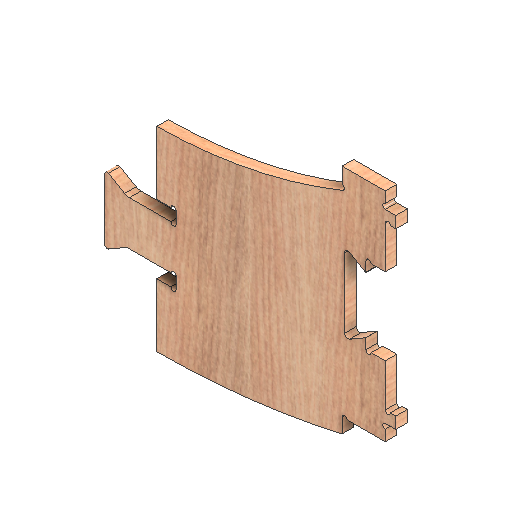
# Autodesk Inventor part: Support C
Saved by Autodesk Inventor 2021 (Build 250183000, 183)
## iProperties
Created: 2020-05-09
Part Number: Support C
Material: Wood (Birch)
Document SubType Name: Modeling
Designer: Dan Wikman
Density: 0.55 g/cm^3
Appearance: Birch - Natural Polished
Mass: 1099.51 g
Surface Area: 2585.2 cm^2
Volume: 1999.1 cm^3
Autodesk Inventor part; units mm, degrees
ref_plane "YZ Plane" through (0, 0, 0) normal (1, 0, 0) x (0, 1, 0)
ref_plane "XZ Plane" through (0, 0, 0) normal (0, 1, 0) x (-1, 0, 0)
ref_plane "XY Plane" through (0, 0, 0) normal (0, 0, 1) x (1, 0, 0)
sketch "CONTOURS" plane through (0, 0, 0) normal (0, 0, 1) x (1, 0, 0)
  arc A0 (167.5054, 852.7989) -> (159.5054, 852.7989) centre (163.5054, 852.7989) ccw
  line L0 (159.5054, 852.7989) -> (95.0246, 852.7989)
  arc A1 (95.0246, 852.7989) -> (87.5246, 850.7893) centre (95.0246, 837.7989) ccw
  line L1 (87.5246, 850.7893) -> (62.3643, 836.263)
  arc A2 (56.3643, 839.7271) -> (62.3643, 836.263) centre (60.3643, 839.7271) ccw
  line L2 (56.3643, 839.7271) -> (56.3643, 934.8707)
  arc A3 (62.3643, 938.3348) -> (56.3643, 934.8707) centre (60.3643, 934.8707) ccw
  line L3 (62.3643, 938.3348) -> (87.5246, 923.8085)
  arc A4 (87.5246, 923.8085) -> (95.0246, 921.7989) centre (95.0246, 936.7989) ccw
  line L4 (95.0246, 921.7989) -> (136.0054, 921.7989)
  line L5 (136.0054, 921.7989) -> (159.5054, 921.7989)
  arc A5 (159.5054, 921.7989) -> (167.5054, 921.7989) centre (163.5054, 921.7989) ccw
  line L6 (167.5054, 921.7989) -> (167.5054, 940.7989)
  arc A6 (167.5054, 940.7989) -> (159.5054, 940.7989) centre (163.5054, 940.7989) ccw
  line L7 (159.5054, 940.7989) -> (137.5054, 940.7989)
  line L8 (137.5054, 940.7989) -> (137.5054, 1039.1352)
  arc A7 (137.5054, 1039.1352) -> (426.0054, 1097.3015) centre (128.2106, 1829.7885) ccw
  arc A8 (426.0054, 1097.3015) -> (426.0054, 1105.3015) centre (426.0054, 1101.3015) ccw
  line L9 (426.0054, 1105.3015) -> (426.0054, 1129.8557)
  line L10 (426.0054, 1129.8557) -> (493.1464, 1129.8556)
  line L11 (493.1464, 1129.8556) -> (493.1464, 1113.0556)
  arc A9 (493.1464, 1113.0556) -> (493.1464, 1105.0556) centre (493.1464, 1109.0556) ccw
  line L12 (493.1464, 1105.0556) -> (509.6464, 1105.0556)
  line L13 (509.6464, 1105.0556) -> (509.6464, 1087.0556)
  line L14 (509.6464, 1087.0556) -> (501.1464, 1087.0556)
  arc A10 (501.1464, 1087.0556) -> (493.1464, 1087.0556) centre (497.1464, 1087.0556) ccw
  line L15 (493.1464, 1087.0556) -> (493.1464, 1020.8556)
  line L16 (493.1464, 1020.8556) -> (471.1464, 1020.8556)
  arc A11 (471.1464, 1020.8556) -> (463.1464, 1020.8556) centre (467.1464, 1020.8556) ccw
  line L17 (463.1464, 1020.8556) -> (463.1464, 1004.6734)
  line L18 (463.1464, 1004.6734) -> (462.9047, 1004.8036)
  line L19 (462.9047, 1004.8036) -> (462.6656, 1004.9385)
  line L20 (462.6656, 1004.9385) -> (437.5054, 1019.4648)
  arc A12 (437.5054, 1019.4648) -> (430.0054, 1015.1347) centre (435.0054, 1015.1347) ccw
  line L21 (430.0054, 1015.1347) -> (430.0054, 906.5765)
  arc A13 (430.0054, 906.5765) -> (437.5054, 902.2464) centre (435.0054, 906.5765) ccw
  line L22 (437.5054, 902.2464) -> (462.6656, 916.7727)
  line L23 (462.6656, 916.7727) -> (462.9047, 916.9076)
  line L24 (462.9047, 916.9076) -> (463.1464, 917.0378)
  line L25 (463.1464, 917.0378) -> (463.1464, 900.8556)
  arc A14 (463.1464, 900.8556) -> (471.1464, 900.8556) centre (467.1464, 900.8556) ccw
  line L26 (471.1464, 900.8556) -> (493.1464, 900.8556)
  line L27 (493.1464, 900.8556) -> (493.1464, 834.6556)
  arc A15 (493.1464, 834.6556) -> (501.1464, 834.6556) centre (497.1464, 834.6556) ccw
  line L28 (501.1464, 834.6556) -> (509.6464, 834.6556)
  line L29 (509.6464, 834.6556) -> (509.6464, 816.6556)
  line L30 (509.6464, 816.6556) -> (493.1464, 816.6556)
  arc A16 (493.1464, 816.6556) -> (493.1464, 808.6556) centre (493.1464, 812.6556) ccw
  line L31 (493.1464, 808.6556) -> (493.1464, 791.8557)
  line L32 (493.1464, 791.8557) -> (434.0054, 791.8557)
  arc A17 (434.0054, 791.8557) -> (426.0054, 791.8557) centre (430.0054, 791.8557) ccw
  line L33 (426.0054, 791.8557) -> (426.0054, 768.8809)
  arc A18 (137.5054, 735.4635) -> (426.0054, 768.8809) centre (133.6317, 2030.9546) ccw
  line L34 (137.5054, 735.4635) -> (137.5054, 833.7989)
  line L35 (137.5054, 833.7989) -> (159.5054, 833.7989)
  arc A19 (159.5054, 833.7989) -> (167.5054, 833.7989) centre (163.5054, 833.7989) ccw
  line L36 (167.5054, 833.7989) -> (167.5054, 852.7989)
  constraints: 74 end point, 40 point on circle, 20 centre point
sketch "LETTERS" plane through (0, 0, 0) normal (0, 0, 1) x (1, 0, 0)
  line L0 (285.7416, 916.5238) -> (285.9594, 916.4912)
  line L1 (285.9594, 916.4912) -> (286.1742, 916.4519)
  line L2 (286.1742, 916.4519) -> (286.386, 916.4061)
  line L3 (286.386, 916.4061) -> (286.5947, 916.3537)
  line L4 (286.5947, 916.3537) -> (286.8003, 916.2951)
  line L5 (286.8003, 916.2951) -> (287.0028, 916.2304)
  line L6 (287.0028, 916.2304) -> (287.2021, 916.1595)
  line L7 (287.2021, 916.1595) -> (287.3982, 916.0828)
  line L8 (287.3982, 916.0828) -> (287.5911, 916.0003)
  line L9 (287.5911, 916.0003) -> (287.7807, 915.9122)
  line L10 (287.7807, 915.9122) -> (287.967, 915.8185)
  line L11 (287.967, 915.8185) -> (288.1499, 915.7195)
  line L12 (288.1499, 915.7195) -> (288.3295, 915.6152)
  line L13 (288.3295, 915.6152) -> (288.5057, 915.5058)
  line L14 (288.5057, 915.5058) -> (288.6784, 915.3914)
  line L15 (288.6784, 915.3914) -> (288.8477, 915.2722)
  line L16 (288.8477, 915.2722) -> (289.0135, 915.1482)
  line L17 (289.0135, 915.1482) -> (289.1757, 915.0197)
  line L18 (289.1757, 915.0197) -> (289.3343, 914.8867)
  line L19 (289.3343, 914.8867) -> (289.4894, 914.7494)
  line L20 (289.4894, 914.7494) -> (289.6408, 914.6079)
  line L21 (289.6408, 914.6079) -> (289.7885, 914.4624)
  line L22 (289.7885, 914.4624) -> (289.9325, 914.3129)
  line L23 (289.9325, 914.3129) -> (290.0728, 914.1596)
  line L24 (290.0728, 914.1596) -> (290.2093, 914.0027)
  line L25 (290.2093, 914.0027) -> (290.3419, 913.8423)
  line L26 (290.3419, 913.8423) -> (290.4708, 913.6784)
  line L27 (290.4708, 913.6784) -> (290.5957, 913.5113)
  line L28 (290.5957, 913.5113) -> (290.7168, 913.3411)
  line L29 (290.7168, 913.3411) -> (290.8339, 913.1679)
  line L30 (290.8339, 913.1679) -> (290.947, 912.9918)
  line L31 (290.947, 912.9918) -> (291.0561, 912.813)
  line L32 (291.0561, 912.813) -> (291.1611, 912.6315)
  line L33 (291.1611, 912.6315) -> (291.2621, 912.4476)
  line L34 (291.2621, 912.4476) -> (291.359, 912.2614)
  line L35 (291.359, 912.2614) -> (291.4517, 912.073)
  line L36 (291.4517, 912.073) -> (291.5402, 911.8825)
  line L37 (291.5402, 911.8825) -> (291.6245, 911.69)
  line L38 (291.6245, 911.69) -> (291.7046, 911.4958)
  line L39 (291.7046, 911.4958) -> (291.7803, 911.2999)
  line L40 (291.7803, 911.2999) -> (291.8518, 911.1024)
  line L41 (291.8518, 911.1024) -> (291.9189, 910.9035)
  line L42 (291.9189, 910.9035) -> (291.9816, 910.7034)
  line L43 (291.9816, 910.7034) -> (292.0399, 910.5021)
  line L44 (292.0399, 910.5021) -> (292.0938, 910.2998)
  line L45 (292.0938, 910.2998) -> (292.1431, 910.0966)
  line L46 (292.1431, 910.0966) -> (292.1879, 909.8927)
  line L47 (292.1879, 909.8927) -> (292.2282, 909.6881)
  line L48 (292.2282, 909.6881) -> (292.2639, 909.4831)
  line L49 (292.2639, 909.4831) -> (292.295, 909.2777)
  line L50 (292.295, 909.2777) -> (292.3214, 909.0721)
  line L51 (292.3214, 909.0721) -> (292.3431, 908.8665)
  line L52 (292.3431, 908.8665) -> (292.3601, 908.6608)
  line L53 (292.3601, 908.6608) -> (292.3724, 908.4554)
  line L54 (292.3724, 908.4554) -> (292.3798, 908.2502)
  line L55 (292.3798, 908.2502) -> (292.3825, 908.0455)
  line L56 (292.3825, 908.0455) -> (292.3802, 907.8414)
  line L57 (292.3802, 907.8414) -> (292.3731, 907.638)
  line L58 (292.3731, 907.638) -> (292.3611, 907.4354)
  line L59 (292.3611, 907.4354) -> (292.3441, 907.2338)
  line L60 (292.3441, 907.2338) -> (292.3221, 907.0333)
  line L61 (292.3221, 907.0333) -> (292.295, 906.834)
  line L62 (292.295, 906.834) -> (292.2629, 906.6361)
  line L63 (292.2629, 906.6361) -> (292.2257, 906.4397)
  line L64 (292.2257, 906.4397) -> (292.1834, 906.2449)
  line L65 (292.1834, 906.2449) -> (292.1361, 906.0518)
  line L66 (292.1361, 906.0518) -> (292.0838, 905.8604)
  line L67 (292.0838, 905.8604) -> (292.0265, 905.6708)
  line L68 (292.0265, 905.6708) -> (291.9645, 905.483)
  line L69 (291.9645, 905.483) -> (291.8977, 905.297)
  line L70 (291.8977, 905.297) -> (291.8263, 905.1128)
  line L71 (291.8263, 905.1128) -> (291.7502, 904.9306)
  line L72 (291.7502, 904.9306) -> (291.6697, 904.7503)
  line L73 (291.6697, 904.7503) -> (291.5847, 904.5721)
  line L74 (291.5847, 904.5721) -> (291.4954, 904.3958)
  line L75 (291.4954, 904.3958) -> (291.4018, 904.2217)
  line L76 (291.4018, 904.2217) -> (291.304, 904.0496)
  line L77 (291.304, 904.0496) -> (291.2021, 903.8797)
  line L78 (291.2021, 903.8797) -> (291.0961, 903.712)
  line L79 (291.0961, 903.712) -> (290.9861, 903.5465)
  line L80 (290.9861, 903.5465) -> (290.8723, 903.3833)
  line L81 (290.8723, 903.3833) -> (290.7547, 903.2224)
  line L82 (290.7547, 903.2224) -> (290.6333, 903.0638)
  line L83 (290.6333, 903.0638) -> (290.5083, 902.9077)
  line L84 (290.5083, 902.9077) -> (290.3797, 902.754)
  line L85 (290.3797, 902.754) -> (290.2476, 902.6027)
  line L86 (290.2476, 902.6027) -> (290.112, 902.454)
  line L87 (290.112, 902.454) -> (289.9732, 902.3078)
  line L88 (289.9732, 902.3078) -> (289.831, 902.1642)
  line L89 (289.831, 902.1642) -> (289.6857, 902.0232)
  line L90 (289.6857, 902.0232) -> (289.5372, 901.8849)
  line L91 (289.5372, 901.8849) -> (289.3857, 901.7493)
  line L92 (289.3857, 901.7493) -> (289.2313, 901.6165)
  line L93 (289.2313, 901.6165) -> (289.0739, 901.4864)
  line L94 (289.0739, 901.4864) -> (288.9138, 901.3592)
  line L95 (288.9138, 901.3592) -> (288.7509, 901.2348)
  line L96 (288.7509, 901.2348) -> (288.5854, 901.1134)
  line L97 (288.5854, 901.1134) -> (288.4173, 900.9949)
  line L98 (288.4173, 900.9949) -> (288.2468, 900.8794)
  line L99 (288.2468, 900.8794) -> (288.0738, 900.7669)
  line L100 (288.0738, 900.7669) -> (287.8984, 900.6575)
  line L101 (287.8984, 900.6575) -> (287.7208, 900.5512)
  line L102 (287.7208, 900.5512) -> (287.5411, 900.448)
  line L103 (287.5411, 900.448) -> (287.3592, 900.348)
  line L104 (287.3592, 900.348) -> (287.1753, 900.2513)
  line L105 (287.1753, 900.2513) -> (286.9894, 900.1578)
  line L106 (286.9894, 900.1578) -> (286.8017, 900.0677)
  line L107 (286.8017, 900.0677) -> (286.6121, 899.9808)
  line L108 (286.6121, 899.9808) -> (286.4209, 899.8974)
  line L109 (286.228, 899.8174) -> (286.0335, 899.7409)
  line L110 (286.0335, 899.7409) -> (285.8375, 899.6679)
  line L111 (285.8375, 899.6679) -> (285.6402, 899.5984)
  line L112 (285.6402, 899.5984) -> (285.4415, 899.5325)
  line L113 (285.4415, 899.5325) -> (285.2415, 899.4703)
  line L114 (285.2415, 899.4703) -> (285.0404, 899.4117)
  line L115 (285.0404, 899.4117) -> (284.8382, 899.3568)
  line L116 (284.8382, 899.3568) -> (284.635, 899.3057)
  line L117 (284.635, 899.3057) -> (284.4308, 899.2583)
  line L118 (284.4308, 899.2583) -> (284.2257, 899.2148)
  line L119 (284.2257, 899.2148) -> (284.0199, 899.1751)
  line L120 (284.0199, 899.1751) -> (283.8133, 899.1394)
  line L121 (283.8133, 899.1394) -> (283.6061, 899.1076)
  line L122 (283.6061, 899.1076) -> (283.3984, 899.0797)
  line L123 (283.3984, 899.0797) -> (283.1902, 899.0559)
  line L124 (283.1902, 899.0559) -> (282.9815, 899.0362)
  line L125 (282.9815, 899.0362) -> (282.7726, 899.0206)
  line L126 (282.7726, 899.0206) -> (282.5634, 899.0091)
  line L127 (282.5634, 899.0091) -> (282.354, 899.0018)
  line L128 (282.354, 899.0018) -> (282.1446, 898.9986)
  line L129 (282.1446, 898.9986) -> (281.9351, 898.9995)
  line L130 (281.9351, 898.9995) -> (281.7257, 899.0046)
  line L131 (281.7257, 899.0046) -> (281.5165, 899.0137)
  line L132 (281.5165, 899.0137) -> (281.3075, 899.0268)
  line L133 (281.3075, 899.0268) -> (281.0987, 899.0439)
  line L134 (281.0987, 899.0439) -> (280.8904, 899.065)
  line L135 (280.8904, 899.065) -> (280.6825, 899.09)
  line L136 (280.6825, 899.09) -> (280.4751, 899.1189)
  line L137 (280.4751, 899.1189) -> (280.2683, 899.1517)
  line L138 (280.2683, 899.1517) -> (280.0623, 899.1883)
  line L139 (280.0623, 899.1883) -> (279.8569, 899.2287)
  line L140 (279.8569, 899.2287) -> (279.6525, 899.2729)
  line L141 (279.6525, 899.2729) -> (279.4489, 899.3208)
  line L142 (279.4489, 899.3208) -> (279.2464, 899.3724)
  line L143 (279.2464, 899.3724) -> (279.0449, 899.4277)
  line L144 (279.0449, 899.4277) -> (278.8446, 899.4866)
  line L145 (278.8446, 899.4866) -> (278.6455, 899.5491)
  line L146 (278.6455, 899.5491) -> (278.4478, 899.6153)
  line L147 (278.4478, 899.6153) -> (278.2514, 899.6849)
  line L148 (278.2514, 899.6849) -> (278.0565, 899.7581)
  line L149 (278.0565, 899.7581) -> (277.8631, 899.8348)
  line L150 (277.8631, 899.8348) -> (277.6714, 899.9149)
  line L151 (277.6714, 899.9149) -> (277.4813, 899.9985)
  line L152 (277.4813, 899.9985) -> (277.2931, 900.0854)
  line L153 (277.2931, 900.0854) -> (277.1067, 900.1757)
  line L154 (277.1067, 900.1757) -> (276.9222, 900.2693)
  line L155 (276.9222, 900.2693) -> (276.7397, 900.3662)
  line L156 (276.7397, 900.3662) -> (276.5594, 900.4664)
  line L157 (276.5594, 900.4664) -> (276.3812, 900.5698)
  line L158 (276.3812, 900.5698) -> (276.2052, 900.6764)
  line L159 (276.2052, 900.6764) -> (276.0316, 900.7861)
  line L160 (276.0316, 900.7861) -> (275.8604, 900.899)
  line L161 (275.8604, 900.899) -> (275.6916, 901.015)
  line L162 (275.6916, 901.015) -> (275.5254, 901.1341)
  line L163 (275.5254, 901.1341) -> (275.3619, 901.2562)
  line L164 (275.3619, 901.2562) -> (275.201, 901.3813)
  line L165 (275.201, 901.3813) -> (275.043, 901.5094)
  line L166 (275.043, 901.5094) -> (274.8878, 901.6405)
  line L167 (274.8878, 901.6405) -> (274.7355, 901.7744)
  line L168 (274.7355, 901.7744) -> (274.5863, 901.9113)
  line L169 (274.5863, 901.9113) -> (274.4402, 902.0509)
  line L170 (274.4402, 902.0509) -> (274.2973, 902.1934)
  line L171 (274.2973, 902.1934) -> (274.1576, 902.3387)
  line L172 (274.1576, 902.3387) -> (274.0213, 902.4868)
  line L173 (274.0213, 902.4868) -> (273.8883, 902.6375)
  line L174 (273.8883, 902.6375) -> (273.7589, 902.791)
  line L175 (273.7589, 902.791) -> (273.633, 902.9471)
  line L176 (273.633, 902.9471) -> (273.5108, 903.1058)
  line L177 (273.5108, 903.1058) -> (273.3923, 903.2671)
  line L178 (273.3923, 903.2671) -> (273.2777, 903.431)
  line L179 (273.2777, 903.431) -> (273.1669, 903.5974)
  line L180 (273.1669, 903.5974) -> (273.06, 903.7664)
  line L181 (273.06, 903.7664) -> (272.9572, 903.9378)
  line L182 (272.9572, 903.9378) -> (272.8585, 904.1116)
  line L183 (272.8585, 904.1116) -> (272.764, 904.2878)
  line L184 (272.764, 904.2878) -> (272.6738, 904.4664)
  line L185 (272.6738, 904.4664) -> (272.5879, 904.6473)
  line L186 (272.5879, 904.6473) -> (272.5065, 904.8306)
  line L187 (272.5065, 904.8306) -> (272.4295, 905.0161)
  line L188 (272.4295, 905.0161) -> (272.3572, 905.2039)
  line L189 (272.3572, 905.2039) -> (272.2895, 905.3938)
  line L190 (272.2895, 905.3938) -> (272.2265, 905.586)
  line L191 (272.2265, 905.586) -> (272.1683, 905.7803)
  line L192 (272.1683, 905.7803) -> (272.115, 905.9766)
  line L193 (272.115, 905.9766) -> (272.0664, 906.1748)
  line L194 (272.0664, 906.1748) -> (272.0226, 906.3747)
  line L195 (272.0226, 906.3747) -> (271.9836, 906.5761)
  line L196 (271.9836, 906.5761) -> (271.9493, 906.7791)
  line L197 (271.9493, 906.7791) -> (271.9198, 906.9833)
  line L198 (271.9198, 906.9833) -> (271.8949, 907.1887)
  line L199 (271.8949, 907.1887) -> (271.8748, 907.3951)
  line L200 (271.8748, 907.3951) -> (271.8594, 907.6024)
  line L201 (271.8594, 907.6024) -> (271.8487, 907.8104)
  line L202 (271.8487, 907.8104) -> (271.8426, 908.019)
  line L203 (271.8426, 908.019) -> (271.8413, 908.2281)
  line L204 (271.8413, 908.2281) -> (271.8445, 908.4375)
  line L205 (271.8445, 908.4375) -> (271.8524, 908.6471)
  line L206 (271.8524, 908.6471) -> (271.8649, 908.8567)
  line L207 (271.8649, 908.8567) -> (271.882, 909.0662)
  line L208 (271.882, 909.0662) -> (271.9037, 909.2754)
  line L209 (271.9037, 909.2754) -> (271.93, 909.4843)
  line L210 (271.93, 909.4843) -> (271.9609, 909.6926)
  line L211 (271.9609, 909.6926) -> (271.9963, 909.9003)
  line L212 (271.9963, 909.9003) -> (272.0363, 910.1071)
  line L213 (272.0363, 910.1071) -> (272.0807, 910.313)
  line L214 (272.0807, 910.313) -> (272.1298, 910.5178)
  line L215 (272.1298, 910.5178) -> (272.1833, 910.7213)
  line L216 (272.1833, 910.7213) -> (272.2412, 910.9235)
  line L217 (272.2412, 910.9235) -> (272.3037, 911.1242)
  line L218 (272.3037, 911.1242) -> (272.3706, 911.3232)
  line L219 (272.3706, 911.3232) -> (272.442, 911.5204)
  line L220 (272.442, 911.5204) -> (272.5179, 911.7157)
  line L221 (272.5179, 911.7157) -> (272.5981, 911.9089)
  line L222 (272.5981, 911.9089) -> (272.6828, 912.0998)
  line L223 (272.6828, 912.0998) -> (272.7718, 912.2884)
  line L224 (272.7718, 912.2884) -> (272.8652, 912.4745)
  line L225 (272.8652, 912.4745) -> (272.9631, 912.6579)
  line L226 (272.9631, 912.6579) -> (273.0652, 912.8386)
  line L227 (273.0652, 912.8386) -> (273.1717, 913.0163)
  line L228 (273.1717, 913.0163) -> (273.2826, 913.191)
  line L229 (273.2826, 913.191) -> (273.3978, 913.3624)
  line L230 (273.3978, 913.3624) -> (273.5172, 913.5305)
  line L231 (273.5172, 913.5305) -> (273.641, 913.6951)
  line L232 (273.641, 913.6951) -> (273.7691, 913.8561)
  line L233 (273.7691, 913.8561) -> (273.9014, 914.0133)
  line L234 (273.9014, 914.0133) -> (274.038, 914.1666)
  line L235 (274.038, 914.1666) -> (274.1788, 914.3158)
  line L236 (274.1788, 914.3158) -> (274.3238, 914.4608)
  line L237 (274.3238, 914.4608) -> (274.4731, 914.6015)
  line L238 (274.4731, 914.6015) -> (274.6265, 914.7377)
  line L239 (274.6265, 914.7377) -> (274.7842, 914.8693)
  line L240 (274.7842, 914.8693) -> (274.946, 914.9961)
  line L241 (274.946, 914.9961) -> (275.112, 915.118)
  line L242 (275.112, 915.118) -> (275.2821, 915.2349)
  line L243 (275.2821, 915.2349) -> (275.4564, 915.3466)
  line L244 (275.4564, 915.3466) -> (275.6348, 915.453)
  line L245 (275.6348, 915.453) -> (275.8173, 915.5538)
  line L246 (275.8173, 915.5538) -> (276.0039, 915.6491)
  line L247 (276.0039, 915.6491) -> (276.1946, 915.7387)
  line L248 (276.1946, 915.7387) -> (276.3894, 915.8223)
  line L249 (276.3894, 915.8223) -> (276.5882, 915.8999)
  line L250 (276.5882, 915.8999) -> (276.7911, 915.9713)
  line L251 (276.7911, 915.9713) -> (276.998, 916.0365)
  line L252 (276.998, 916.0365) -> (277.2089, 916.0951)
  line L253 (277.2089, 916.0951) -> (277.4238, 916.1472)
  line L254 (277.4238, 916.1472) -> (277.6428, 916.1925)
  line L255 (286.4209, 899.8974) -> (286.228, 899.8174)
  constraints: 512 end point
extrude "Extrusion1" add sketch "CONTOURS" along normal blind 18
body "Solid1"
